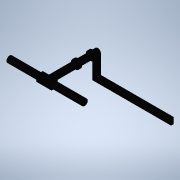
# Autodesk Inventor part: Lenkung_vorne
Saved by Autodesk Inventor 2020 (Build 240168000, 168)
## iProperties
Created: 2020-02-25
Part Number: Lenkung_vorne
Material: Generisch
Document SubType Name: Modeling
Designer: Stefan
Density: 1 g/cm^3
Appearance: Vorgabe
Mass: 351.719 g
Surface Area: 703.447 cm^2
Volume: 351.719 cm^3
Author: Stefan
Autodesk Inventor part; units mm, degrees
ref_plane "YZ Plane" through (0, 0, 0) normal (1, 0, 0) x (0, 1, 0)
ref_plane "XZ Plane" through (0, 0, 0) normal (0, 1, 0) x (-1, 0, 0)
ref_plane "XY Plane" through (0, 0, 0) normal (0, 0, 1) x (1, 0, 0)
sketch "Skizze1" plane through (0, 0, 0) normal (0, 0, 1) x (1, 0, 0)
  circle A0 centre (0, 0) radius 12.45
  dimension "d0" = 24.9
  constraints: 1 centre point, 1 coincident
  measures "d0" diameter of A0
extrude "Extrusion1" add sketch "Skizze1" along normal blind 50
sketch "Skizze2" plane through (0, 0, 50) normal (0, 0, 1) x (1, 0, 0)
  circle A0 centre (0, 0) radius 17.5
  dimension "d3" = 35
  constraints: 1 centre point, 1 coincident
  measures "d3" diameter of A0
extrude "Extrusion2" add sketch "Skizze2" along normal blind 10
sketch "Skizze3" plane through (0, 0, 0) normal (0, 0, -1) x (-1, 0, 0)
  circle A0 centre (0, 0) radius 17.5
  dimension "d6" = 35
  constraints: 1 centre point, 1 coincident
  measures "d6" diameter of A0
extrude "Extrusion3" add sketch "Skizze3" along normal blind 10
sketch "Skizze4" plane through (0, 0, -10) normal (0, 0, -1) x (-1, 0, 0)
  circle A0 centre (0, 0) radius 12.5
  dimension "d9" = 25
  constraints: 1 centre point, 1 coincident
  measures "d9" diameter of A0
extrude "Extrusion4" add sketch "Skizze4" along normal blind 10
sketch "Skizze5" plane through (0, 0, 60) normal (0, 0, 1) x (1, 0, 0)
  circle A0 centre (0, 0) radius 12.5
  dimension "d12" = 25
  constraints: 1 centre point, 1 coincident
  measures "d12" diameter of A0
extrude "Extrusion5" add sketch "Skizze5" along normal blind 100
sketch "Skizze6" plane through (0, 0, -20) normal (0, 0, -1) x (-1, 0, 0)
  line L0 (-12.5, 0) -> (12.5, 0)
  line L1 (12.5, 0) -> (12.5, -100)
  line L2 (12.5, -100) -> (-12.5, -100)
  line L3 (-12.5, -100) -> (-12.5, 0)
  circle A0 centre (0, 0) radius 17.5 projected
  arc A1 (12.5, 0) -> (-12.5, 0) centre (0, 0) ccw
  line L4 (0, 0) -> (12.5, 0) construction
  line L5 (0, 0) -> (-12.5, 0) construction
  dimension "d15" = 25
  dimension "d16" = 12.5
  dimension "d17" = 0
  dimension "d18" = 100
  dimension "d19" = 180
  constraints: 12 end point, 2 parallel, 2 point on circle, 1 centre point, 1 coincident, 1 horizontal, 1 perpendicular
  measures "d15" distance of L0.start L0.end
  measures "d16" distance from line of L1 point (0, 0)
  measures "d17" distance from line of point (0, 0) L0
  measures "d18" distance of L0.end L1.end
  measures "d19" angle of L5 L4
extrude "Extrusion6" add sketch "Skizze6" along normal blind 10 contours A1 L0 | L0 L1 A0 L3 | A0 L1 L2 L3
sketch "Skizze8" plane through (0, 0, -30) normal (0, 0, -1) x (-1, 0, 0)
  line L0 (-12.5, -100) -> (-302.5, -100)
  line L1 (-302.5, -100) -> (-302.5, -75)
  line L2 (-302.5, -75) -> (-12.5, -75)
  line L3 (-12.5, -75) -> (-12.5, -100)
  line L4 (-12.5, 0) -> (-12.5, -100) projected
  line L5 (-12.5, -100) -> (12.5, -100) projected
  point P0 (0, 0)
  dimension "d23" = 25
  dimension "d24" = 0
  dimension "d26" = 290
  dimension "d29" = 0
  constraints: 8 end point, 2 parallel, 1 horizontal, 1 perpendicular
  measures "d23" distance of L0.end L1.end
  measures "d24" distance between parallel lines of L5 L0
  measures "d26" distance of L0.start L0.end
  measures "d29" distance between parallel lines of L3 L4
extrude "Extrusion7" add sketch "Skizze8" against normal blind 10
sketch "Skizze9" plane through (0, 0, -20) normal (0, 0, 1) x (1, 0, 0)
  circle A0 centre (292.5, -87.5) radius 6
  line L0 (302.5, -100) -> (302.5, -75) projected
  line L1 (-12.5, -100) -> (302.5, -100) projected
  point P0 (0, 0)
  dimension "d30" = 12
  dimension "d31" = 10
  dimension "d32" = 12.5
  constraints: 1 centre point
  measures "d30" diameter of A0
  measures "d31" distance from line of L0 A0.centre
  measures "d32" distance from line of L1 A0.centre
extrude "Extrusion8" cut sketch "Skizze9" against normal up to surface (10 mm away)
sketch "Skizze10" plane through (0, 0, 160) normal (0, 0, 1) x (1, 0, 0)
  line L0 (150, -12.5) -> (-150, -12.5)
  line L1 (-150, -12.5) -> (-150, 12.5)
  line L2 (-150, 12.5) -> (150, 12.5)
  line L3 (150, 12.5) -> (150, -12.5)
  point P0 (0, 0)
  dimension "d35" = 25
  dimension "d36" = 12.5
  dimension "d37" = 300
  dimension "d38" = 150
  constraints: 8 end point, 2 parallel, 1 horizontal, 1 perpendicular
  measures "d35" distance of L0.end L1.end
  measures "d36" distance from line of L0 point (0, 0)
  measures "d37" distance of L0.start L0.end
  measures "d38" distance from line of L1 point (0, 0)
extrude "Extrusion9" add sketch "Skizze10" along normal blind 25
sketch "Skizze11" plane through (150, -12.5, 160) normal (1, 0, 0) x (0, 0, -1)
  line L0 (0, 0) -> (-25, 0) projected
  line L1 (-25, 25) -> (-25, 0) projected
  line L2 (0, 0) -> (-25, 0)
  line L3 (-25, 0) -> (-25, 25)
  line L4 (-25, 25) -> (0, 25)
  line L5 (0, 25) -> (0, 0)
  circle A0 centre (-12.5, 12.5) radius 12.5
  point P0 (160, 12.5)
  point P1 (-25, 12.5)
  point P2 (-12.5, 25)
  point P3 (0, 12.5)
  point P4 (-12.5, 0)
  constraints: 8 end point, 2 parallel, 1 centre point, 1 horizontal, 1 perpendicular, 1 tangent
extrude "Extrusion10" cut sketch "Skizze11" against normal blind 120 contours L0 A0 L5 | L0 L1 A0 | A0 L4 L5 | L1 L4 A0
sketch "Skizze12" plane through (-150, -12.5, 160) normal (-1, 0, 0) x (0, 0, 1)
  line L0 (0, 25) -> (25, 25) projected
  line L1 (0, 0) -> (25, 0)
  line L2 (25, 0) -> (25, 25)
  line L3 (25, 25) -> (0, 25)
  line L4 (0, 25) -> (0, 0)
  circle A0 centre (12.5, 12.5) radius 12.5
  point P0 (-160, 12.5)
  point P1 (12.5, 25)
  point P2 (25, 12.5)
  point P3 (12.5, 0)
  point P4 (0, 12.5)
  constraints: 8 end point, 2 parallel, 1 centre point, 1 horizontal, 1 perpendicular
extrude "Extrusion11" cut sketch "Skizze12" against normal blind 120 contours L0 A0 L4 | L0 L2 A0 | A0 L1 L4 | L2 L1 A0
